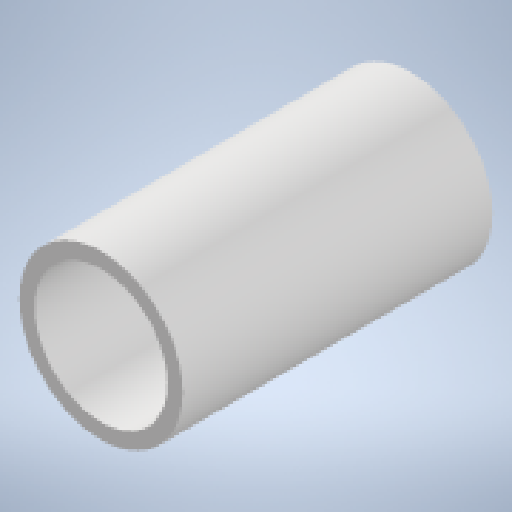
# Autodesk Inventor part: TuboC
Saved by Autodesk Inventor 2023.1 (Build 271208000, 208)
## iProperties
Created: 2022-08-29
Part Number: TuboC
Material: Generic
Document SubType Name: Modeling
Designer: Daniel Peña
Density: 1 g/cm^3
Appearance: Default
Author: Daniel Peña
Autodesk Inventor part; units mm, degrees
ref_plane "YZ Plane" through (0, 0, 0) normal (1, 0, 0) x (0, 1, 0)
ref_plane "XZ Plane" through (0, 0, 0) normal (0, 1, 0) x (-1, 0, 0)
ref_plane "XY Plane" through (0, 0, 0) normal (0, 0, 1) x (1, 0, 0)
sketch "Sketch1" plane through (0, 0, 0) normal (0, 1, 0) x (-1, 0, 0)
  line L0 (6.3, 33.95) -> (4.3, 33.95)
  line L1 (4.3, 33.95) -> (4.3, -6.45)
  line L2 (4.3, -6.45) -> (6.3, -6.45)
  line L3 (6.3, -6.45) -> (6.3, 33.95)
  line L4 (-4.35, 3.5833) -> (-4.35, -8.1167)
  point P0 (0, 0)
  dimension "d0" = 2
  dimension "d1" = 40.4
  dimension "d2" = 21.3
  constraints: 10 end point, 2 parallel, 1 horizontal, 1 perpendicular, 1 vertical
  measures "d0" distance of L1.end L2.end
  measures "d1" distance of L2.end L0.start
  measures "d2" diameter of L3 L4
revolve "Revolution1" add sketch "Sketch1" angle 360 about axis through (4.35, 0, 3.5833) along (0, 0, -1)
body "Solid1"
